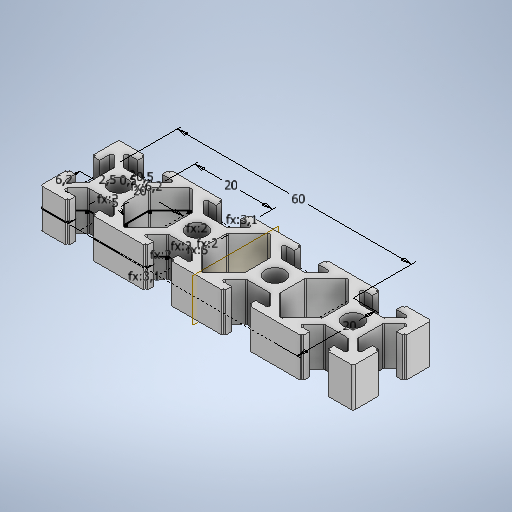
# Autodesk Inventor part: Peça7
Saved by Autodesk Inventor 2025.2 (Build 292293000, 293)
## iProperties
Created: 2025-04-04
Part Number: Peça7
Material: Genérico
Document SubType Name: Modelagem
Designer: kenay
Density: 1 g/cm^3
Appearance: Padrão
Sheet Metal Rule: Padrão_mm
Author: kenay
Autodesk Inventor part; units mm, degrees
ref_plane "YZ Plane" through (0, 0, 0) normal (1, 0, 0) x (0, 1, 0)
ref_plane "XZ Plane" through (0, 0, 0) normal (0, 1, 0) x (-1, 0, 0)
ref_plane "XY Plane" through (0, 0, 0) normal (0, 0, 1) x (1, 0, 0)
sketch "Esboço1" plane through (0, 0, 0) normal (0, 1, 0) x (-1, 0, 0)
  line L0 (10, 10) -> (30, 10) construction
  line L1 (30, 10) -> (30, -10) construction
  line L2 (30, -10) -> (10, -10) construction
  line L3 (10, -10) -> (10, 10) construction
  line L4 (10, 10) -> (30, -10) construction
  line L5 (30, 10) -> (10, -10) construction
  line L6 (20, -10) -> (20, 10) construction
  line L7 (25.9536, -7.1464) -> (23.4536, -4.6464)
  line L8 (25.6, -8) -> (23.1, -8)
  arc A0 (25.6, -8) -> (25.9536, -7.1464) centre (25.6, -7.5) ccw
  line L9 (23.1, -9.5) -> (23.1, -8)
  line L10 (23.6, -9.5) -> (23.1, -9.5)
  line L11 (23.6, -10) -> (23.6, -9.5)
  line L12 (30, -10) -> (23.6, -10) construction
  line L13 (30, -10) -> (20, -10) construction
  line L14 (30, -10) -> (30, -3.6) construction
  line L15 (29.5, -3.1) -> (28, -3.1)
  line L16 (29.5, -3.1) -> (29.5, -3.6)
  line L17 (29.5, -3.6) -> (30, -3.6)
  line L18 (28, -3.1) -> (28, -5.6)
  line L19 (27.1464, -5.9536) -> (24.6464, -3.4536)
  arc A1 (24.5, -3.1) -> (24.6464, -3.4536) centre (25, -3.1) ccw
  line L20 (30, 0) -> (20, 0) construction
  arc A2 (27.1464, -5.9536) -> (28, -5.6) centre (27.5, -5.6) ccw
  arc A3 (29.5, -10) -> (30, -9.5) centre (29.5, -9.5) ccw
  line L21 (29.5, -10) -> (23.6, -10)
  line L22 (30, -9.5) -> (30, -3.6)
  circle A4 centre (20, 0) radius 2.5
  line L23 (29.5, 3.1) -> (28, 3.1)
  line L24 (28, 3.1) -> (28, 5.6)
  line L25 (25.6, 8) -> (23.1, 8)
  line L26 (23.1, 8) -> (23.1, 9.5)
  line L27 (23.1, 9.5) -> (23.6, 9.5)
  line L28 (23.6, 9.5) -> (23.6, 10)
  line L29 (29.5, 3.1) -> (29.5, 3.6)
  line L30 (29.5, 3.6) -> (30, 3.6)
  line L31 (27.1464, 5.9536) -> (24.6464, 3.4536)
  line L32 (25.9536, 7.1464) -> (23.4536, 4.6464)
  arc A5 (28, 5.6) -> (27.1464, 5.9536) centre (27.5, 5.6) ccw
  arc A6 (30, 9.5) -> (29.5, 10) centre (29.5, 9.5) ccw
  line L33 (30, 9.5) -> (30, 3.6)
  line L34 (29.5, 10) -> (23.6, 10)
  arc A7 (25.9536, 7.1464) -> (25.6, 8) centre (25.6, 7.5) ccw
  line L35 (24.5, -3.1) -> (24.5, 3.1)
  arc A8 (24.6464, 3.4536) -> (24.5, 3.1) centre (25, 3.1) ccw
  arc A9 (23.1, 4.5) -> (23.4536, 4.6464) centre (23.1, 5) ccw
  line L36 (23.1, 4.5) -> (16.9, 4.5)
  line L37 (16.5464, 4.6464) -> (14.0464, 7.1464)
  arc A10 (16.5464, 4.6464) -> (16.9, 4.5) centre (16.9, 5) ccw
  line L38 (16.9, 8) -> (14.4, 8)
  line L39 (16.9, 8) -> (16.9, 9.5)
  line L40 (16.9, 9.5) -> (16.4, 9.5)
  line L41 (16.4, 9.5) -> (16.4, 10)
  line L42 (10, 10) -> (16.4, 10)
  arc A11 (14.4, 8) -> (14.0464, 7.1464) centre (14.4, 7.5) ccw
  line L43 (16.5464, -4.6464) -> (14.0464, -7.1464)
  line L44 (16.9, -8) -> (16.9, -9.5)
  line L45 (16.9, -9.5) -> (16.4, -9.5)
  line L46 (16.4, -9.5) -> (16.4, -10)
  line L47 (16.4, -10) -> (10, -10)
  line L48 (16.9, -8) -> (14.4, -8)
  arc A12 (14.0464, -7.1464) -> (14.4, -8) centre (14.4, -7.5) ccw
  line L49 (23.1, -4.5) -> (16.9, -4.5)
  arc A13 (23.4536, -4.6464) -> (23.1, -4.5) centre (23.1, -5) ccw
  arc A14 (16.9, -4.5) -> (16.5464, -4.6464) centre (16.9, -5) ccw
  line L50 (15.3536, 3.4536) -> (10.3536, 8.4536)
  arc A15 (15.5, 3.1) -> (15.3536, 3.4536) centre (15, 3.1) ccw
  line L51 (15.5, -3.1) -> (15.5, 3.1)
  line L52 (15.3536, -3.4536) -> (10.3536, -8.4536)
  arc A16 (15.3536, -3.4536) -> (15.5, -3.1) centre (15, -3.1) ccw
  arc A17 (0, -2.5) -> (0, 2.5) centre (0, 0) ccw
  line L53 (30, -10) -> (-30, -10) construction
  line L54 (-30, -10) -> (-30, 10) construction
  line L55 (-30, 10) -> (30, 10) construction
  line L56 (30, 10) -> (30, -10) construction
  line L57 (0, -10) -> (0, 10) construction
  line L58 (4.5, -3.1) -> (4.5, 3.1)
  line L59 (9.6464, -8.4536) -> (4.6464, -3.4536)
  line L60 (9.6464, 8.4536) -> (4.6464, 3.4536)
  arc A18 (10.3536, 8.4536) -> (9.6464, 8.4536) centre (10, 8.1) ccw
  arc A19 (4.6464, 3.4536) -> (4.5, 3.1) centre (5, 3.1) ccw
  arc A20 (4.5, -3.1) -> (4.6464, -3.4536) centre (5, -3.1) ccw
  arc A21 (9.6464, -8.4536) -> (10.3536, -8.4536) centre (10, -8.1) ccw
  line L61 (10, 10) -> (3.6, 10)
  line L62 (3.6, 10) -> (3.6, 9.5)
  line L63 (3.6, 9.5) -> (3.1, 9.5)
  line L64 (3.1, 9.5) -> (3.1, 8)
  line L65 (3.1, 8) -> (5.1574, 8)
  line L66 (5.5109, 7.1464) -> (3.0109, 4.6464)
  arc A22 (5.5109, 7.1464) -> (5.1574, 8) centre (5.1574, 7.5) ccw
  line L67 (2.6574, 4.5) -> (0, 4.5)
  arc A23 (2.6574, 4.5) -> (3.0109, 4.6464) centre (2.6574, 5) ccw
  line L68 (0, 4.5) -> (0, 2.5)
  line L69 (0, -2.5) -> (0, -4.5)
  line L70 (3.0109, -4.6464) -> (5.5109, -7.1464)
  line L71 (0, -4.5) -> (2.6574, -4.5)
  arc A24 (3.0109, -4.6464) -> (2.6574, -4.5) centre (2.6574, -5) ccw
  line L72 (10, -10) -> (3.6, -10)
  line L73 (3.6, -9.5) -> (3.6, -10)
  line L74 (3.6, -9.5) -> (3.1, -9.5)
  line L75 (3.1, -9.5) -> (3.1, -8)
  line L76 (3.1, -8) -> (5.1574, -8)
  arc A25 (5.1574, -8) -> (5.5109, -7.1464) centre (5.1574, -7.5) ccw
  line L77 (20, -4.5) -> (20, -2.5)
  line L78 (20, 2.5) -> (20, 4.5)
  point P0 (24.5, 0)
  point P1 (0, 0)
  point P2 (20, 0)
  point P3 (0, 0)
  point P4 (4.2609, -5.8964)
  dimension "d0" = 20
  dimension "d7" = 0.5
  dimension "d8" = 2
  dimension "d17" = 5
  dimension "d18" = 6.2
  dimension "d23" = 2
  dimension "d25" = 0.5
  dimension "d26" = 2.5
  dimension "d27" = 6.2
  dimension "d29" = 20
  dimension "d30" = 5
  dimension "d31" = 60
  dimension "d32" = 20
  dimension "d33" = 2
  dimension "d34" = 3.1
  dimension "d35" = 2
  dimension "d36" = 2
  dimension "d37" = 3.1
  dimension "d38" = 2
  constraints: 158 end point, 52 point on circle, 49 tangent, 40 equal length, 26 centre point, 20 equal radius, 18 perpendicular, 17 point on line, 16 horizontal, 13 midpoint, 13 vertical, 8 collinear, 7 parallel, 2 coincident, 1 horizontal alignment, 6 other
  measures "d0" distance between parallel lines of L3 L1
  measures "d7" distance of L9.start L10.start
  measures "d8" distance between parallel lines of L12 L8
  measures "d17" diameter of A4
  measures "d18" distance between parallel lines of L15 L23
  measures "d23" distance edge to line of A4 L35
  measures "d25" radius of A0
  measures "d26" distance of L15.end L18.end
  measures "d27" distance between parallel lines of L44 L9
  measures "d29" distance of point (0, 0) point (20, 0)
  measures "d30" diameter of A17
  measures "d31" distance of L1.end L53.end
  measures "d32" distance of L53.end L54.end
  measures "d33" distance edge to line of A17 L58
  measures "d34" distance between parallel lines of L57 L64
  measures "d35" distance between parallel lines of L66 L60
  measures "d36" distance from line of L59 point (4.261, -5.896)
  measures "d37" distance between parallel lines of L57 L75
  measures "d38" distance from line of L69.start L71
extrude "Extrusão1" add sketch "Esboço1" along normal mid plane 10 contours L49 A14 L43 A12 L48 L44 L45 L46 L47 L72 L73 L74 L75 L76 A25 L70 A24 L71 L69 A17 L68 L67 A23 L66 A22 L65 L64 L63 L62 L61 L42 L41 L40 L39 L38 A11 L37 A10 L36 L78 A4 L77
pattern_linear "Padrão retangular1" count 3 spacing 20 along (1, 0, 0) of "Extrusão1"
ref_plane "Plano de trabalho1" through (10, -5, -4.5) normal (1, 0, 0) x (0, 0, -1)
extrude "Extrusão2" add sketch "Esboço1" along normal mid plane 10 contours L7 A13 L49 L77 A4 L78 L36 A9 L32 A7 L25 L26 L27 L28 L34 A6 L33 L30 L29 L23 L24 A5 L31 A8 L35 A1 L19 A2 L18 L15 L16 L17 L22 A3 L21 L11 L10 L9 L8 A0
mirror "Espelhar3" about plane through (10, -5, -4.5) normal (1, 0, 0) of "Extrusão2"
equation "\"d23\" = d8"
equation "\"d27\" = d18"
equation "\"d30\" = d17"
equation "\"d33\" = d23"
equation "\"d34\" = 0.5 * d18"
equation "\"d35\" = d23"
equation "\"Raio_vergadura\" = Espessura"
equation "\"Largura_alívio_de_vergadura\" = Espessura"
equation "\"Profundidade_alívio_de_vergadura\" = 0.5 * Espessura"
equation "\"Tamanho_alívio_de_dobra\" = 4 * Espessura"
equation "\"Remanescente_mínimo\" = 2 * Espessura"
equation "\"Raiodetransição\" = Raio_vergadura"
equation "\"Tamanho_de_raio_de_Jacobi\" = Raio_vergadura"
equation "\"TamanhoFolga\" = Espessura"
equation "\"Espessura\" = 0.5"
